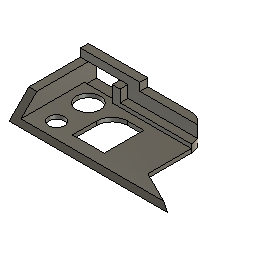
test-wall-holls (Autodesk Fusion 360 design; units mm, degrees)
Autodesk Fusion 360 part; units mm, degrees
sketch "Sketch1" plane through (0, 0, 0) normal (0, 0, 1) x (1, 0, 0) in component "test"
  line L0 (-10, 10) -> (5, 10)
  line L1 (5, 10) -> (5, 0)
  line L2 (5, 0) -> (-10, 0)
  line L3 (-10, 0) -> (-10, 10)
  line L4 (5, 0) -> (10, 0)
  line L5 (10, 0) -> (5, 2.5)
  dimension "d1" = 15
  dimension "d2" = 10
  constraint horizontal L0
  constraint vertical L1
  constraint horizontal L2
  constraint vertical L3
  constraint perpendicular L1 L4
  constraint coincident L1 L5.end
  measures "d1" distance of L0.start L0.end
  measures "d2" distance of L0.start L2.end
extrude "Extrude1" add sketch "Sketch1" along normal blind 0.5 in component "test"
sketch "Sketch2" plane through (0, 0, 0.5) normal (0, 0, 1) x (-1, 0, 0) in component "test"
  line L0 (10, 0) -> (-10, 0)
  line L1 (-5, -2.5) -> (-5, -10)
  line L2 (-5, -10) -> (10, -10)
  line L3 (10, -10) -> (10, 0)
  line L4 (10, -10) -> (9, -10)
  line L5 (9, -10) -> (9, 0)
  line L6 (9, 0) -> (10, 0)
  line L7 (10, 0) -> (10, -10)
  line L8 (-5, -10) -> (5, -10)
  line L9 (5, -10) -> (5, -8)
  line L10 (5, -8) -> (-5, -8)
  line L11 (-5, -8) -> (-5, -10)
  line L12 (-10, 0) -> (-5, -2.5)
  constraint horizontal L4
  constraint vertical L5
  constraint horizontal L6
  constraint vertical L7
  constraint coincident L0 L5.end
  constraint coincident L2.end L3.start
  constraint horizontal L8
  constraint vertical L9
  constraint horizontal L10
  constraint vertical L11
  constraint coincident L1.end L2.start
extrude "Extrude2" add sketch "Sketch2" along normal blind 2 contours L0 L2 L3 L4 L5 L6 L7 | L1 L2 L8 L9 L10 L11 in component "test"
sketch "Sketch3" plane through (0, 0, 2.5) normal (0, 0, 1) x (-1, 0, 0) in component "test"
  line L0 (-5, -8) -> (-5, -10)
  line L1 (-5, -10) -> (5, -10)
  line L2 (5, -10) -> (5, -8)
  line L3 (5, -8) -> (-5, -8)
  line L4 (-5, -8) -> (4, -8)
  line L5 (4, -8) -> (4, -9)
  line L6 (4, -9) -> (-5, -9)
  line L7 (-5, -9) -> (-5, -8)
  constraint horizontal L4
  constraint vertical L5
  constraint horizontal L6
  constraint vertical L7
  constraint coincident L0.start L3.end
extrude "Extrude3" cut sketch "Sketch3" against normal blind 1.5 contours L0 L3 L4 L5 L6 L7 in component "test"
sketch "Sketch4" plane through (0, 0, 0.5) normal (0, 0, 1) x (-1, 0, 0) in component "test"
  line L0 (5, -8) -> (5, -10)
  line L1 (5, -10) -> (9, -10)
  line L2 (9, -10) -> (9, 0)
  line L3 (9, 0) -> (-10, 0)
  line L4 (-5, -2.5) -> (-5, -8)
  line L5 (-5, -8) -> (5, -8)
  line L6 (0, -7) -> (4, -7)
  line L7 (4, -7) -> (4, -2)
  line L8 (4, -2) -> (0, -2)
  line L9 (0, -2) -> (0, -7)
  circle A0 centre (6.5, -6.5) radius 1.5
  circle A1 centre (6.5, -2.5) radius 1
  line L10 (-10, 0) -> (-5, -2.5)
  dimension "d9" = 3
  dimension "d10" = 2
  constraint horizontal L6
  constraint vertical L7
  constraint horizontal L8
  constraint vertical L9
  measures "d9" diameter of A0
  measures "d10" diameter of A1
extrude "Extrude4" cut sketch "Sketch4" against normal through all contours L6 L7 L8 L9 | A0 | A1 in component "test"
sketch "Sketch5" plane through (0, 0, 2.5) normal (0, 0, 1) x (-1, 0, 0) in component "test"
  line L0 (10, 0) -> (9, 0)
  line L1 (9, 0) -> (9, -10)
  line L2 (9, -10) -> (10, -10)
  line L3 (10, -10) -> (10, 0)
  line L4 (10, -10) -> (2.5, -10)
  line L5 (2.5, -10) -> (2.5, -9)
  line L6 (2.5, -9) -> (10, -9)
  line L7 (10, -9) -> (10, -10)
  constraint horizontal L4
  constraint vertical L5
  constraint horizontal L6
  constraint vertical L7
  constraint coincident L2.end L3.start
extrude "Extrude5" add sketch "Sketch5" along normal blind 1 contours L1 L2 L3 L4 L6 L7 | L1 L4 L5 L6 in component "test"
chamfer "Chamfer1" distance 2.5 angle 45 1 edges at (-9.5, 0, 2.5) in component "test"
fillet "Fillet1" radius 2 1 edges at (5, 10, 1.25) in component "test"
fillet "Fillet2" radius 2 1 edges at (-4, 7, 0.25) in component "test"
sketch "Sketch6" plane through (0, 0, 0.5) normal (0, 0, 1) x (-1, 0, 0) in component "test"
  line L0 (9, -0.5) -> (-9, -0.5)
  line L1 (-9, -0.5) -> (-5, -2.5)
  line L2 (-5, -2.5) -> (-5, -8)
  line L3 (-5, -8) -> (5, -8)
  line L4 (5, -8) -> (5, -10)
  line L5 (5, -10) -> (9, -10)
  line L6 (9, -10) -> (9, -0.5)
  line L7 (0, -2) -> (4, -2)
  line L8 (4, -2) -> (4, -5)
  arc A0 (2, -7) -> (4, -5) centre (2, -5) ccw
  line L9 (2, -7) -> (0, -7)
  line L10 (0, -7) -> (0, -2)
  circle A1 centre (6.5, -6.5) radius 1.5
  circle A2 centre (6.5, -2.5) radius 1
  line L11 (5, -8.5) -> (9, -8.5)
  line L12 (9, -8.5) -> (9, -10)
  line L13 (9, -10) -> (5, -10)
  line L14 (5, -10) -> (5, -8.5)
  constraint horizontal L11
  constraint vertical L12
  constraint horizontal L13
  constraint vertical L14
  constraint coincident L5.end L6.start
  constraint coincident L4 L11.start
extrude "Extrude6" cut sketch "Sketch6" against normal blind 0.3 contours L4 L5 L6 L11 L12 L13 L14 in component "test"
component "test" placed x (1, 0, 0) y (0, 1, 0) z (0, 0, 1) at (0, 0, 0)
